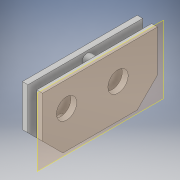
# Autodesk Inventor part: gabetrain
Saved by Autodesk Inventor 2017 (Build 210142000, 142)
## iProperties
Created: 2017-04-12
Part Number: gabetrain
Material: Generic
Document SubType Name: Modeling
Designer: User
Density: 1 g/cm^3
Appearance: Default
Author: User
Autodesk Inventor part; units mm, degrees
ref_plane "YZ Plane" through (0, 0, 0) normal (1, 0, 0) x (0, 1, 0)
ref_plane "XZ Plane" through (0, 0, 0) normal (0, 1, 0) x (-1, 0, 0)
ref_plane "XY Plane" through (0, 0, 0) normal (0, 0, 1) x (1, 0, 0)
sketch "Sketch1" plane through (0, 0, 0) normal (1, 0, 0) x (0, 1, 0)
  line L0 (0, 0) -> (9.6932, 0)
  line L1 (9.6932, 0) -> (9.6932, -18.0074)
  line L2 (9.6932, -18.0074) -> (0, -18.0074)
  line L3 (0, -18.0074) -> (0, 0)
  constraints: 8 end point, 2 parallel, 1 horizontal, 1 perpendicular
extrude "Extrusion1" add sketch "Sketch1" along normal blind 3.175
chamfer "Chamfer1" distance 3.175 angle 45 1 edges at (1.5875, 0, 0)
chamfer "Chamfer2" distance 3.175 angle 45 1 edges at (1.5875, 0, -18.0074)
hole "Hole1" at (3.175, 5.775, -3.7524) direction (-1, 0, 0) diameter 3.175 depth 3.175 tip angle 118
hole "Hole2" at (3.175, 5.3978, -11.8179) direction (-1, 0, 0) diameter 3.175 depth 3.175 tip angle 118
sketch "Sketch2" plane through (0, 9.6932, 0) normal (0, 0, 1) x (1, 0, 0)
  line L0 (0, 0) -> (3.175, 0) projected
  line L1 (1.5875, 0) -> (0.8676, 0)
  line L2 (0.8676, 0) -> (0.8676, -11.3231)
  line L3 (0.8676, -11.3231) -> (1.5875, -11.3231)
  line L4 (1.5875, -11.3231) -> (1.5875, 0)
  line L5 (1.5875, 0) -> (2.2609, 0)
  line L6 (2.2609, 0) -> (2.2609, -11.3231)
  line L7 (2.2609, -11.3231) -> (1.5875, -11.3231)
  line L8 (1.5875, -11.3231) -> (1.5875, 0)
  point P0 (0, -9.6932)
  constraints: 16 end point, 4 parallel, 2 horizontal, 2 perpendicular, 1 midpoint, 1 point on line
extrude "Extrusion2" cut sketch "Sketch2" against normal blind 254
ref_plane "Work Plane1" through (3.2004, 0, 0) normal (1, 0, 0) x (0, 0, -1)
sketch "Sketch3" plane through (3.2004, 0, 0) normal (1, 0, 0) x (0, 0, -1)
  circle A0 centre (9.2621, 8.5805) radius 0.766
  point P0 (0, 0)
  constraints: 1 centre point
extrude "Extrusion3" add sketch "Sketch3" against normal blind 3.175
sketch "Sketch4" plane through (3.175, 0, 0) normal (1, 0, 0) x (0, 0, -1)
  circle A0 centre (4.9587, 2.3914) radius 0.8506
  point P0 (0, 0)
  constraints: 1 centre point
extrude "Extrusion4" add sketch "Sketch4" against normal blind 3.175
thicken "Thicken1" operation add thickness 0.0254 both sides no extend neighbours yes toward (-1, 0, 0) faces at (3.2004, 8.8685, -9.0418)
sketch "Sketch5" plane through (3.175, 3.175, -18.0074) normal (1, 0, 0) x (0, 0, -1)
  circle A0 centre (-2.6542, -0.8404) radius 1.0945
  point P0 (-18.0074, -3.175)
  constraints: 1 centre point
extrude "Extrusion5" add sketch "Sketch5" against normal blind 3.175
body "Solid1"
